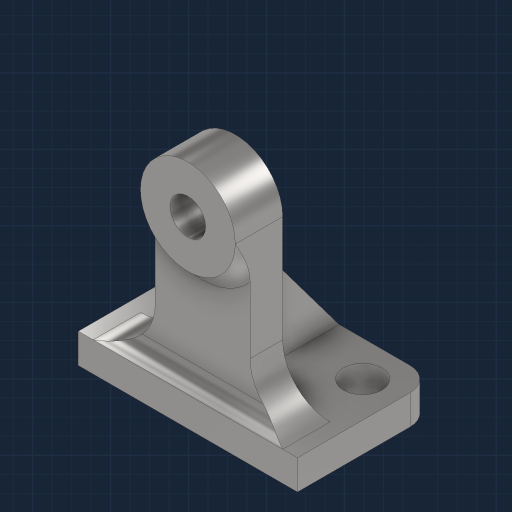
# Autodesk Inventor part: 02-bracket
Saved by Autodesk Inventor 2024 (Build 280153000, 153)
## iProperties
Created: 2025-03-09
Part Number: 02-bracket
Material: Steel, Carbon
Document SubType Name: Modeling
Designer: DuctopwH
Density: 7.85 g/cm^3
Appearance: Semi-Polished
Author: DuctopwH
Autodesk Inventor part; units mm, degrees
ref_plane "YZ Plane" through (0, 0, 0) normal (1, 0, 0) x (0, 1, 0)
ref_plane "XZ Plane" through (0, 0, 0) normal (0, 1, 0) x (-1, 0, 0)
ref_plane "XY Plane" through (0, 0, 0) normal (0, 0, 1) x (1, 0, 0)
sketch "Sketch2" plane through (0, 0, 0) normal (0, 0, 1) x (1, 0, 0)
  circle A0 centre (0, 62) radius 16
  line L0 (0, 62) -> (0, 0) construction
  line L1 (-16, 62) -> (-16, 0)
  line L2 (-16, 0) -> (0, 0)
  line L3 (16, 62) -> (16, 0)
  line L4 (16, 0) -> (0, 0)
  point P0 (16, 62)
  dimension "d0" = 32
  dimension "d1" = 62
  constraints: 10 end point, 3 vertical, 2 symmetric about line, 1 perpendicular, 3 other
  measures "d1" distance from line of L2 L0.start
extrude "Extrusion1" add sketch "Sketch2" along normal blind 11
sketch "Sketch3" plane through (-16, 0, 0) normal (0, -1, 0) x (1, 0, 0)
  line L0 (53, -30) -> (-21, -30)
  line L1 (-21, -30) -> (-21, 16)
  line L2 (-21, 16) -> (53, 16)
  line L3 (53, 16) -> (53, -30)
  line L4 (53, -30) -> (-21, 16) construction
  line L5 (-21, -30) -> (53, 16) construction
  line L6 (0, 11) -> (32, 11) projected
  line L7 (0, 0) -> (32, 0) projected
  point P0 (16, 0)
  point P1 (16, -7)
  point P2 (16, 0)
  dimension "d4" = 5
  dimension "d5" = 74
  dimension "d6" = 46
  constraints: 12 end point, 3 midpoint, 2 parallel, 1 horizontal, 1 perpendicular, 1 vertical alignment
  measures "d4" distance between parallel lines of L6 L2
  measures "d5" distance between parallel lines of L3 L1
  measures "d6" distance of L0.end L1.end
extrude "Extrusion2" add sketch "Sketch3" against normal blind 10
sketch "Sketch4" plane through (0, 0, 0) normal (1, 0, 0) x (0, 1, 0)
  line L0 (10, 16) -> (10, -30) construction
  line L1 (10, -30) -> (50, 0)
  line L2 (10, 0) -> (62, 0) construction
  point P0 (0, 0)
  dimension "d9" = 40
  constraints: 2 end point, 1 point on line
  measures "d9" horizontal distance of L0.end L1.end
extrude "Rib1" add sketch "Sketch4" along normal mid plane 10 rib yes fills toward (29.97, -14.96) open curves L1
sketch "Sketch5" plane through (0, 0, 11) normal (0, 0, 1) x (1, 0, 0)
  circle A0 centre (0, 62) radius 16
  arc A1 (16, 62) -> (-16, 62) centre (0, 62) ccw projected
  point P0 (0, 0)
  constraints: 2 concentric, 1 centre point
extrude "Extrusion3" add sketch "Sketch5" along normal up to surface (5 mm away)
sketch "Sketch6" plane through (0, 62, 16) normal (0, 0, 1) x (1, 0, 0)
  circle A0 centre (0, 0) radius 16 projected
  point P0 (0, -62)
  constraints: 1 coincident
hole "Hole1" at (0, 62, 16) direction (0, 0, -1) diameter 12 end through all
sketch "Sketch7" plane through (-16, 10, 0) normal (0, 1, 0) x (1, 0, 0)
  line L0 (-21, 30) -> (-21, -16) projected
  line L1 (11, 30) -> (-21, 30) projected
  point P0 (16, 0)
  point P1 (-9, 18)
  dimension "d25" = 12
  dimension "d26" = 12
  measures "d25" distance from line of L0 point (-9, 18)
  measures "d26" distance from line of L1 point (-9, 18)
hole "Hole2" at (-25, 10, -18) direction (0, -1, 0) diameter 13 end through all
pattern_linear "Rectangular Pattern1" count 2 spacing 50 along (1, 0, 0) of "Hole2"
fillet "Fillet1" radius 16 2 edges at (-16, 10, 5.5) (16, 10, 5.5)
fillet "Fillet2" radius 5 4 edges at (0, 46, 11) (24, 10, 11) (0, 10, 11) (-24, 10, 11)
fillet "Fillet3" radius 8 2 edges at (-37, 5, -30) (37, 5, -30)
body "Solid1"
